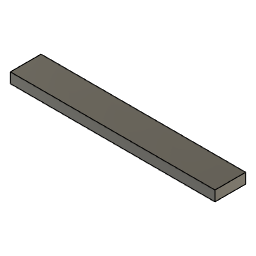
教壇[特にいらないかな] (Autodesk Fusion 360 design; units mm, degrees)
Autodesk Fusion 360 part; units mm, degrees
sketch "スケッチ1" plane through (0, 0, 0) normal (0, 1, 0) x (1, 0, 0)
  line L0 (0, 0) -> (-6000, 0)
  line L1 (-6000, 0) -> (-6000, -300)
  line L2 (-6000, -300) -> (0, -300)
  line L3 (0, -300) -> (0, 0)
  dimension "d1" = 6000
  dimension "d2" = 300
  constraint horizontal L0
  constraint vertical L1
  constraint horizontal L2
  constraint vertical L3
  constraint coincident L0.start L3.end
  measures "d1" distance of L0.start L0.end
  measures "d2" distance of L0.start L2.end
extrude "押し出し1" add sketch "スケッチ1" along normal blind 900
